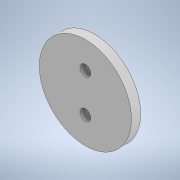
# Autodesk Inventor part: 轴端挡圈
Saved by Autodesk Inventor 2020 (Build 240168000, 168)
## iProperties
Created: 2021-06-17
Part Number: 轴端挡圈
Material: 常规
Document SubType Name: Modeling
Designer: dell
Density: 1 g/cm^3
Appearance: 默认
Author: dell
Autodesk Inventor part; units mm, degrees
ref_plane "YZ Plane" through (0, 0, 0) normal (1, 0, 0) x (0, 1, 0)
ref_plane "XZ Plane" through (0, 0, 0) normal (0, 1, 0) x (-1, 0, 0)
ref_plane "XY Plane" through (0, 0, 0) normal (0, 0, 1) x (1, 0, 0)
sketch "草图1" plane through (0, 0, 0) normal (0, 0, 1) x (1, 0, 0)
  circle A0 centre (0, 0) radius 30
  line L0 (0, -42) -> (0, 42) construction
  circle A1 centre (0, 12.5) radius 3.5
  circle A2 centre (0, -12.5) radius 3.5
  line L1 (-42, 0) -> (42, 0) construction
  dimension "d0" = 60
  dimension "d1" = 7
  dimension "d2" = 7
  dimension "d3" = 25
  constraints: 3 centre point, 2 point on line, 1 coincident, 1 symmetric about line
  measures "d0" diameter of A0
  measures "d1" diameter of A1
  measures "d2" diameter of A2
  measures "d3" distance of A2.centre A1.centre
extrude "拉伸1" add sketch "草图1" along normal blind 6
